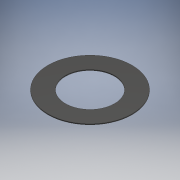
# Autodesk Inventor part: ポリスラ12-24 0.25mm
Saved by Autodesk Inventor 2017.3 (Build 213256000, 256)
## iProperties
Part Number: ポリスラ12-24 0.25mm
Material: アセタール樹脂、黒
Document SubType Name: Modeling
Designer: 原知也
Mass: 0.106323 g
Surface Area: 6.26748 cm^2
Volume: 0.0746128 cm^3
Density: 1.425 g/cm^3
Appearance: 滑らか - 黒
Author: 原知也
Autodesk Inventor part; units mm, degrees
ref_plane "YZ Plane" through (0, 0, 0) normal (1, 0, 0) x (0, 1, 0)
ref_plane "XZ Plane" through (0, 0, 0) normal (0, 1, 0) x (-1, 0, 0)
ref_plane "XY Plane" through (0, 0, 0) normal (0, 0, 1) x (1, 0, 0)
sketch "スケッチ1" plane through (0, 0, 0) normal (0, 0, 1) x (1, 0, 0)
  circle A0 centre (0, 0) radius 7
  circle A1 centre (0, 0) radius 12
  dimension "d0" = 14
  dimension "d1" = 24
  constraints: 2 centre point, 2 coincident
  measures "d0" diameter of A0
  measures "d1" diameter of A1
extrude "押し出し1" add sketch "スケッチ1" along normal blind 0.25
